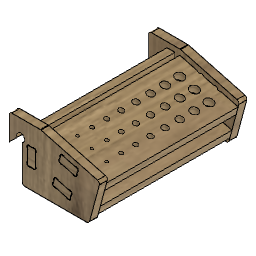
drillbox (Autodesk Fusion 360 design; units mm, degrees)
Autodesk Fusion 360 part; units mm, degrees
note: some values were not read from the file. Set by a fixed rule: which sketch regions a step uses.
sketch "Sketch1" plane through (0, 0, 0) normal (0, 1, 0) x (1, 0, 0) in component "Left"
  line L0 (-26.4881, -75.7327) -> (-26.4881, -48.7327)
  line L1 (-26.4881, -48.7327) -> (-11.4881, -63.7327)
  line L2 (-26.4881, -48.7327) -> (3.3546, -48.7327) construction
  line L3 (-11.4881, -63.7327) -> (-11.4881, -78.7327)
  line L4 (-11.4881, -78.7327) -> (-23.4881, -78.7327)
  line L5 (-11.4881, -78.7327) -> (-11.4881, -16.7327)
  line L6 (-8.4881, -13.7327) -> (-5.4881, -13.7327)
  line L7 (-11.4881, -78.7327) -> (9.1169, -78.7327)
  line L8 (9.8934, -78.6304) -> (74.2289, -61.3918)
  line L9 (9.5119, -78.7327) -> (86.2734, -78.7327) construction
  line L10 (76.3502, -57.7175) -> (65.1603, -15.9562)
  line L11 (62.2625, -13.7327) -> (-5.4881, -13.7327)
  line L12 (64.5645, -13.7327) -> (3.3222, -30.1425)
  arc A0 (74.2289, -61.3918) -> (76.3502, -57.7175) centre (73.4525, -58.494) ccw
  arc A1 (9.1169, -78.7327) -> (9.8934, -78.6304) centre (9.1169, -75.7327) ccw
  arc A2 (-26.4881, -75.7327) -> (-23.4881, -78.7327) centre (-23.4881, -75.7327) ccw
  arc A3 (-8.4881, -13.7327) -> (-11.4881, -16.7327) centre (-8.4881, -16.7327) ccw
  arc A4 (65.1603, -15.9562) -> (62.2625, -13.7327) centre (62.2625, -16.7327) ccw
  point P0 (-26.4881, -78.7327)
  point P1 (-11.4881, -13.7327)
  point P2 (77.1267, -60.6153)
  dimension "d2" = 30
  dimension "d3" = 45
  dimension "d4" = 15
  dimension "d5" = 65
  dimension "d6" = 6
  dimension "d7" = 21
  dimension "d8" = 70
  dimension "d9" = 15
  dimension "d17" = 48.5365
  dimension "d18" = 3
  constraint vertical L0
  constraint horizontal L2
  constraint vertical L3
  constraint perpendicular L0 L4
  constraint perpendicular L2 L5
  constraint perpendicular L5 L6
  constraint perpendicular L3 L7
  constraint horizontal L9
  constraint perpendicular L8 L10
  constraint parallel L6 L11
  constraint parallel L8 L12
  constraint coincident P2 L8
  constraint coincident P2 L10
  constraint tangent L8 A0
  constraint tangent L10 A0
  constraint coincident L9.start L8
  constraint coincident L9.start L7
  constraint tangent L8 A1
  constraint tangent L7 A1
  constraint equal A0 A1
  constraint coincident P0 L0
  constraint coincident P0 L4
  constraint tangent L0 A2
  constraint tangent L4 A2
  constraint equal A0 A2
  constraint coincident P1 L5
  constraint coincident P1 L6
  constraint tangent L5 A3
  constraint tangent L6 A3
  constraint equal A0 A3
  constraint coincident L12.start L11
  constraint coincident L12.start L10
  constraint tangent L11 A4
  constraint tangent L10 A4
  constraint equal A0 A4
  measures "d2" distance of P0 L0.end
  measures "d3" angle of L1 L2
  measures "d4" distance of L0 L1.end
  measures "d5" distance of L3.end P1
  measures "d6" distance of P1 L6.end
  measures "d7" distance of L3.end L9.start
  measures "d8" distance of L9.start P2
  measures "d9" angle of L8 L9
  measures "d17" distance of L8 L12
  measures "d18" radius of A0
extrude "Extrude1" add sketch "Sketch1" along normal blind 9 makes body 1 in component "Left"
sketch "Sketch2" plane through (0, 9, 0) normal (0, 1, 0) x (-1, 0, 0) in component "Deckel"
  line L0 (23.4881, 78.7327) -> (-9.1169, 78.7327)
  line L1 (-9.8934, 78.6304) -> (-74.2289, 61.3918)
  line L2 (-62.2625, 13.7327) -> (8.4881, 13.7327)
  line L3 (11.4881, 16.7327) -> (11.4881, 63.7327)
  line L4 (11.4881, 63.7327) -> (26.4881, 48.7327)
  line L5 (26.4881, 48.7327) -> (26.4881, 75.7327)
  line L6 (-75.5738, 54.8198) -> (-9.1169, 72.6268)
  line L7 (-9.1169, 78.7327) -> (-9.1169, 13.7327) construction
  line L8 (-75.5738, 54.8198) -> (-73.2444, 46.1264)
  line L9 (-73.2444, 46.1264) -> (-6.7876, 63.9335)
  line L10 (-6.7876, 63.9335) -> (-9.1169, 72.6268)
  line L11 (-76.3502, 57.7175) -> (-65.1603, 15.9562)
  arc A0 (-9.1169, 78.7327) -> (-9.8934, 78.6304) centre (-9.1169, 75.7327) ccw
  arc A1 (-74.2289, 61.3918) -> (-76.3502, 57.7175) centre (-73.4525, 58.494) ccw
  arc A2 (-65.1603, 15.9562) -> (-62.2625, 13.7327) centre (-62.2625, 16.7327) ccw
  arc A3 (8.4881, 13.7327) -> (11.4881, 16.7327) centre (8.4881, 16.7327) ccw
  arc A4 (26.4881, 75.7327) -> (23.4881, 78.7327) centre (23.4881, 75.7327) ccw
  line L12 (-76.3502, 57.7175) -> (-65.1603, 15.9562)
  dimension "d12" = 6
  dimension "d14" = 9
  constraint parallel L1 L6
  constraint coincident L0.end L7.start
  constraint coincident L2 L7.end
  constraint perpendicular L2 L7
  constraint coincident L6.end L7
  constraint perpendicular L6 L8
  constraint perpendicular L8 L9
  constraint parallel L8 L10
  constraint collinear L8 L12
  measures "d12" distance of L1 L6
  measures "d14" distance of L6.start L8.end
extrude "Extrude2" add sketch "Sketch2" along normal blind 150 separate body contours L6 L8 L9 L10 L11 L12 makes body 2 in component "Deckel"
ref_plane "WorkPlane1" through (41.1807, 84, 59.3766) normal (0, 1, 0) x (0, 0, 1) in component "Deckel"
mirror "MirrorComponent1" about plane through (0, 0, 0) normal (0, 0, 1) of bodies 1 makes body 3 in component "Right"
sketch "Sketch3" plane through (0, 9, 0) normal (0, 1, 0) x (-1, 0, 0) in component "Boden"
  line L0 (23.4881, 78.7327) -> (-9.1169, 78.7327)
  arc A0 (-9.1169, 78.7327) -> (-9.8934, 78.6304) centre (-9.1169, 75.7327) ccw
  line L1 (-9.8934, 78.6304) -> (-74.2289, 61.3918)
  arc A1 (-74.2289, 61.3918) -> (-76.3502, 57.7175) centre (-73.4525, 58.494) ccw
  line L2 (-76.3502, 57.7175) -> (-65.1603, 15.9562)
  arc A2 (-65.1603, 15.9562) -> (-62.2625, 13.7327) centre (-62.2625, 16.7327) ccw
  line L3 (-62.2625, 13.7327) -> (8.4881, 13.7327)
  arc A3 (8.4881, 13.7327) -> (11.4881, 16.7327) centre (8.4881, 16.7327) ccw
  line L4 (11.4881, 16.7327) -> (11.4881, 63.7327)
  line L5 (11.4881, 63.7327) -> (26.4881, 48.7327)
  line L6 (26.4881, 48.7327) -> (26.4881, 75.7327)
  arc A4 (26.4881, 75.7327) -> (23.4881, 78.7327) centre (23.4881, 75.7327) ccw
  line L7 (-76.3502, 57.7175) -> (-65.1603, 15.9562)
  line L8 (-62.2625, 13.7327) -> (8.4881, 13.7327)
  line L9 (-76.3502, 57.7175) -> (-62.9511, 7.7115) construction
  line L10 (8.4881, 13.7327) -> (-75.9622, 13.7327) construction
  line L11 (-6.7876, 63.9335) -> (-9.1169, 72.6268) construction
  line L12 (-73.2444, 46.1264) -> (-6.7876, 63.9335) construction
  line L13 (-64.5645, 13.7327) -> (1.8923, 31.5397) construction
  line L14 (-66.1174, 19.5282) -> (-68.4468, 28.2215)
  line L15 (-6.7876, 63.9335) -> (-6.7876, 18.0069) construction
  line L16 (-66.1174, 19.5282) -> (-6.7876, 35.4256)
  line L17 (-6.7876, 35.4256) -> (-9.1169, 44.1189)
  line L18 (-9.1169, 44.1189) -> (-68.4468, 28.2215)
  dimension "d22" = 9
  constraint coincident A1.end L2.start
  constraint tangent A1 L9
  constraint parallel L2 L9
  constraint coincident L3.end A3.start
  constraint tangent A3 L10
  constraint parallel L8 L10
  constraint coincident L9 L13.start
  constraint coincident L10 L13.start
  constraint coincident L2 L14.start
  constraint coincident L2 L14.end
  constraint coincident L11.start L12.end
  constraint vertical L15
  constraint coincident L15 L16.end
  constraint perpendicular L7 L16
  constraint perpendicular L14 L18
  measures "d22" distance of L14.start L14.end
extrude "Extrude1'" add sketch "Sketch3" along normal blind 150 separate body contours L2 L7 L14 L16 L17 L18 makes body 4 in component "Boden"
mirror "MirrorComponent2" about plane through (0, 0, 0) normal (0, 0, 1) of bodies 1 makes body 5 in component "Left(Mirror)"
sketch "Sketch1 (2)" plane through (0, 9, 0) normal (0, 1, 0) x (-1, 0, 0) in component "Hinten"
  line L0 (23.4881, 78.7327) -> (-9.1169, 78.7327)
  arc A0 (-9.1169, 78.7327) -> (-9.8934, 78.6304) centre (-9.1169, 75.7327) ccw
  line L1 (-9.8934, 78.6304) -> (-74.2289, 61.3918)
  arc A1 (-74.2289, 61.3918) -> (-76.3502, 57.7175) centre (-73.4525, 58.494) ccw
  line L2 (-76.3502, 57.7175) -> (-65.1603, 15.9562)
  arc A2 (-65.1603, 15.9562) -> (-62.2625, 13.7327) centre (-62.2625, 16.7327) ccw
  line L3 (-62.2625, 13.7327) -> (8.4881, 13.7327)
  arc A3 (8.4881, 13.7327) -> (11.4881, 16.7327) centre (8.4881, 16.7327) ccw
  line L4 (11.4881, 16.7327) -> (11.4881, 63.7327)
  line L5 (11.4881, 63.7327) -> (26.4881, 48.7327)
  line L6 (26.4881, 48.7327) -> (26.4881, 75.7327)
  arc A4 (26.4881, 75.7327) -> (23.4881, 78.7327) centre (23.4881, 75.7327) ccw
  line L7 (5.4881, 19.7327) -> (-3.5119, 19.7327)
  line L8 (-3.5119, 19.7327) -> (-3.5119, 72.7327)
  line L9 (-3.5119, 72.7327) -> (5.4881, 72.7327)
  line L10 (5.4881, 72.7327) -> (5.4881, 19.7327)
  dimension "d26" = 9
  dimension "d27" = 6
  dimension "d28" = 6
  dimension "d29" = 6
  constraint horizontal L7
  constraint vertical L8
  constraint horizontal L9
  constraint vertical L10
  measures "d26" distance of L7.start L7.end
  measures "d27" distance of L3 L7
  measures "d28" distance of L4 L10
  measures "d29" distance of L0 L9
extrude "Extrude1''" add sketch "Sketch1 (2)" along normal blind 150 separate body contours L7 L8 L9 L10 makes body 6 in component "Hinten"
sketch "Sketch1 (3)" plane through (0, 9, 0) normal (0, -1, 0) x (1, 0, 0) in component "Deckel"
  line L0 (6.7876, 63.9335) -> (73.2444, 46.1264)
  line L1 (73.2444, 46.1264) -> (75.5738, 54.8198)
  line L2 (75.5738, 54.8198) -> (9.1169, 72.6268)
  line L3 (9.1169, 72.6268) -> (6.7876, 63.9335)
  line L4 (30.3567, 57.6182) -> (32.6861, 66.3115)
  line L5 (52.0046, 61.1351) -> (49.6752, 52.4418)
  line L6 (49.6752, 52.4418) -> (30.3567, 57.6182)
  line L7 (52.0046, 61.1351) -> (32.6861, 66.3115)
  line L8 (7.9522, 68.2802) -> (31.5214, 61.9648) construction
  line L9 (50.8399, 56.7884) -> (74.4091, 50.4731) construction
  dimension "d32" = 20
  constraint coincident L0 L4.start
  constraint coincident L2 L4.end
  constraint perpendicular L2 L4
  constraint coincident L2 L5.start
  constraint coincident L0 L5.end
  constraint perpendicular L0 L5
  constraint perpendicular L4 L6
  constraint midpoint L3 L8.start
  constraint midpoint L4 L8.end
  constraint midpoint L5 L9.start
  constraint midpoint L1 L9.end
  constraint equal L8 L9
  measures "d32" distance of L4.end L5.start
extrude "Extrude1'''" add sketch "Sketch1 (3)" along normal blind 9 contours L0 L2 L4 L5 L6 L7 bodies 2 in component "Deckel"
sketch "Sketch2 (1)" plane through (0, 159, 0) normal (0, 1, 0) x (-1, 0, 0) in component "Deckel"
  line L0 (-73.2444, 46.1264) -> (-6.7876, 63.9335)
  line L1 (-6.7876, 63.9335) -> (-9.1169, 72.6268)
  line L2 (-9.1169, 72.6268) -> (-75.5738, 54.8198)
  line L3 (-75.5738, 54.8198) -> (-73.2444, 46.1264)
  line L4 (-52.0046, 61.1351) -> (-49.6752, 52.4418)
  line L5 (-30.3567, 57.6182) -> (-32.6861, 66.3115)
  line L6 (-52.0046, 61.1351) -> (-32.6861, 66.3115)
  line L7 (-49.6752, 52.4418) -> (-30.3567, 57.6182)
  line L8 (-50.8399, 56.7884) -> (-74.4091, 50.4731) construction
  line L9 (-31.5214, 61.9648) -> (-7.9522, 68.2802) construction
  dimension "d35" = 20
  constraint coincident L2 L4.start
  constraint coincident L0 L4.end
  constraint perpendicular L0 L4
  constraint coincident L0 L5.start
  constraint coincident L2 L5.end
  constraint perpendicular L2 L5
  constraint midpoint L4 L8.start
  constraint midpoint L3 L8.end
  constraint midpoint L5 L9.start
  constraint midpoint L1 L9.end
  constraint equal L8 L9
  measures "d35" distance of L4.start L5.end
extrude "Extrude2'" add sketch "Sketch2 (1)" along normal blind 9 contours L0 L2 L4 L5 L6 L7 bodies 2 in component "Deckel"
sketch "Sketch3 (2)" plane through (0, 0, 0) normal (0, 1, 0) x (1, 0, 0) in component "Left"
  line L0 (49.6752, -52.4418) -> (52.0046, -61.1351)
  line L1 (52.0046, -61.1351) -> (32.6861, -66.3115)
  line L2 (32.6861, -66.3115) -> (30.3567, -57.6182)
  line L3 (30.3567, -57.6182) -> (49.6752, -52.4418)
  line L4 (30.3567, -57.6182) -> (49.6752, -52.4418)
  line L5 (49.6752, -52.4418) -> (52.0046, -61.1351)
  line L6 (52.0046, -61.1351) -> (32.6861, -66.3115)
  line L7 (32.6861, -66.3115) -> (30.3567, -57.6182)
  constraint coincident L2.end L3.start
  constraint coincident L0.start L3.end
  constraint coincident L0.end L1.start
  constraint coincident L1.end L2.start
extrude "Extrude3" cut sketch "Sketch3 (2)" along normal blind 9 bodies 1 in component "Left"
sketch "Sketch4" plane through (0, 9, 0) normal (0, -1, 0) x (1, 0, 0) in component "Boden"
  line L0 (9.1169, 44.1189) -> (6.7876, 35.4256)
  line L1 (6.7876, 35.4256) -> (66.1174, 19.5282)
  line L2 (66.1174, 19.5282) -> (68.4468, 28.2215)
  line L3 (68.4468, 28.2215) -> (9.1169, 44.1189)
  line L4 (49.6752, 52.4418) -> (52.0046, 61.1351) construction
  line L5 (52.0046, 61.1351) -> (42.5483, 25.8435) construction
  line L6 (42.5483, 25.8435) -> (44.8776, 34.5369)
  line L7 (25.5591, 39.7133) -> (44.8776, 34.5369)
  line L8 (25.5591, 39.7133) -> (23.2298, 31.0199)
  line L9 (23.2298, 31.0199) -> (42.5483, 25.8435)
  dimension "d40" = 20
  constraint coincident L4.end L5.start
  constraint coincident L1 L5.end
  constraint perpendicular L1 L5
  constraint coincident L5 L6.end
  constraint coincident L3 L6.end
  constraint coincident L3 L7.start
  constraint perpendicular L6 L7
  constraint coincident L1 L8.end
  constraint perpendicular L1 L8
  measures "d40" distance of L6.end L7.start
extrude "Extrude2''" add sketch "Sketch4" along normal blind 9 contours L1 L3 L6 L7 L8 L9 bodies 4 in component "Boden"
sketch "Sketch5" plane through (0, 159, 0) normal (0, 1, 0) x (-1, 0, 0) in component "Boden"
  line L0 (-6.7876, 35.4256) -> (-9.1169, 44.1189)
  line L1 (-9.1169, 44.1189) -> (-68.4468, 28.2215)
  line L2 (-68.4468, 28.2215) -> (-66.1174, 19.5282)
  line L3 (-66.1174, 19.5282) -> (-6.7876, 35.4256)
  line L4 (-52.0046, 61.1351) -> (-49.6752, 52.4418)
  line L5 (-52.0046, 61.1351) -> (-42.5483, 25.8435) construction
  line L6 (-44.8776, 34.5369) -> (-42.5483, 25.8435)
  line L7 (-42.5483, 25.8435) -> (-23.2298, 31.0199)
  line L8 (-23.2298, 31.0199) -> (-25.5591, 39.7133)
  line L9 (-25.5591, 39.7133) -> (-44.8776, 34.5369)
  dimension "d43" = 20
  constraint coincident L4.start L5.start
  constraint coincident L3 L5.end
  constraint perpendicular L3 L5
  constraint coincident L5 L6.start
  constraint coincident L1 L6.start
  constraint perpendicular L5 L7
  constraint coincident L1 L8.end
  constraint perpendicular L1 L8
  measures "d43" distance of L5.end L7.end
extrude "Extrude3'" add sketch "Sketch5" along normal blind 9 contours L1 L3 L6 L7 L8 L9 bodies 4 in component "Boden"
sketch "Sketch4 (2)" plane through (0, 0, 0) normal (0, 1, 0) x (1, 0, 0) in component "Left"
  line L0 (25.5591, -39.7133) -> (23.2298, -31.0199)
  line L1 (23.2298, -31.0199) -> (42.5483, -25.8435)
  line L2 (42.5483, -25.8435) -> (44.8776, -34.5369)
  line L3 (44.8776, -34.5369) -> (25.5591, -39.7133)
  line L4 (25.5591, -39.7133) -> (44.8776, -34.5369)
  line L5 (44.8776, -34.5369) -> (42.5483, -25.8435)
  line L6 (42.5483, -25.8435) -> (23.2298, -31.0199)
  line L7 (23.2298, -31.0199) -> (25.5591, -39.7133)
  constraint perpendicular L4 L5
  constraint parallel L4 L6
  constraint parallel L5 L7
  constraint coincident L2.end L3.start
  constraint perpendicular L2 L4
  constraint coincident L0.start L3.end
extrude "Extrude4" cut sketch "Sketch4 (2)" along normal blind 9 bodies 1 in component "Left"
sketch "Sketch2 (2)" plane through (0, 9, 0) normal (0, -1, 0) x (1, 0, 0) in component "Hinten"
  line L0 (3.5119, 72.7327) -> (-5.4881, 72.7327)
  line L1 (-5.4881, 72.7327) -> (-5.4881, 19.7327)
  line L2 (-5.4881, 19.7327) -> (3.5119, 19.7327)
  line L3 (3.5119, 19.7327) -> (3.5119, 72.7327)
  line L4 (-5.4881, 56.2327) -> (3.5119, 56.2327)
  line L5 (3.5119, 56.2327) -> (3.5119, 36.2327)
  line L6 (3.5119, 36.2327) -> (-5.4881, 36.2327)
  line L7 (-5.4881, 36.2327) -> (-5.4881, 56.2327)
  line L8 (-0.9881, 56.2327) -> (-0.9881, 72.7327) construction
  line L9 (-0.9881, 36.2327) -> (-0.9881, 19.7327) construction
  dimension "d48" = 9
  dimension "d49" = 20
  constraint horizontal L4
  constraint vertical L5
  constraint horizontal L6
  constraint vertical L7
  constraint coincident L1 L4.start
  constraint midpoint L4 L8.start
  constraint midpoint L0 L8.end
  constraint midpoint L6 L9.start
  constraint midpoint L2 L9.end
  constraint equal L8 L9
  measures "d48" distance of L4.start L4.end
  measures "d49" distance of L4.start L6.end
extrude "Extrude2'''" add sketch "Sketch2 (2)" along normal blind 9 contours L1 L3 L4 L5 L6 L7 bodies 6 in component "Hinten"
sketch "Sketch3 (3)" plane through (0, 159, 0) normal (0, 1, 0) x (-1, 0, 0) in component "Hinten"
  line L0 (5.4881, 72.7327) -> (-3.5119, 72.7327)
  line L1 (-3.5119, 72.7327) -> (-3.5119, 19.7327)
  line L2 (-3.5119, 19.7327) -> (5.4881, 19.7327)
  line L3 (5.4881, 19.7327) -> (5.4881, 72.7327)
  line L4 (-3.5119, 56.2327) -> (5.4881, 56.2327)
  line L5 (5.4881, 56.2327) -> (5.4881, 36.2327)
  line L6 (5.4881, 36.2327) -> (-3.5119, 36.2327)
  line L7 (-3.5119, 36.2327) -> (-3.5119, 56.2327)
  line L8 (0.9881, 72.7327) -> (0.9881, 56.2327) construction
  line L9 (0.9881, 36.2327) -> (0.9881, 19.7327) construction
  dimension "d52" = 9
  dimension "d53" = 20
  constraint horizontal L4
  constraint vertical L5
  constraint horizontal L6
  constraint vertical L7
  constraint coincident L1 L4.start
  constraint midpoint L0 L8.start
  constraint midpoint L4 L8.end
  constraint midpoint L6 L9.start
  constraint midpoint L2 L9.end
  constraint equal L8 L9
  measures "d52" distance of L4.start L4.end
  measures "d53" distance of L4.start L6.end
extrude "Extrude3''" add sketch "Sketch3 (3)" along normal blind 9 contours L1 L3 L4 L5 L6 L7 bodies 6 in component "Hinten"
sketch "Sketch5 (2)" plane through (0, 0, 0) normal (0, 1, 0) x (1, 0, 0) in component "Left"
  line L0 (-5.4881, -36.2327) -> (3.5119, -36.2327)
  line L1 (3.5119, -36.2327) -> (3.5119, -56.2327)
  line L2 (3.5119, -56.2327) -> (-5.4881, -56.2327)
  line L3 (-5.4881, -56.2327) -> (-5.4881, -36.2327)
extrude "Extrude5" cut sketch "Sketch5 (2)" along normal blind 9 bodies 1 in component "Left"
sketch "Sketch3 (4)" plane through (18.7674, 0, 70.041) normal (0.258819, 0, 0.965926) x (0, 1, 0) in component "Deckel"
  line L0 (9, -34.4097) -> (9, -58.8103)
  line L1 (9, -58.8103) -> (159, -58.8103)
  line L2 (159, -58.8103) -> (159, -34.4097)
  line L3 (159, -34.4097) -> (168, -34.4097)
  line L4 (168, -34.4097) -> (168, -14.4097)
  line L5 (168, -14.4097) -> (159, -14.4097)
  line L6 (159, -14.4097) -> (159, 9.9909)
  line L7 (159, 9.9909) -> (9, 9.9909)
  line L8 (9, 9.9909) -> (9, -14.4097)
  line L9 (9, -14.4097) -> (0, -14.4097)
  line L10 (0, -14.4097) -> (0, -34.4097)
  line L11 (0, -34.4097) -> (9, -34.4097)
  line L12 (0, -24.4097) -> (168, -24.4097) construction
  line L13 (9, -41.61) -> (159, -41.61) construction
  line L14 (9, -7.2094) -> (159, -7.2094) construction
  line L15 (48.2855, -24.4097) -> (48.2855, -7.2094) construction
  line L16 (53.6322, -7.2094) -> (53.6322, 9.9909) construction
  line L17 (66.3625, -24.4097) -> (66.3625, -41.61) construction
  line L18 (72.4731, -41.61) -> (72.4731, -58.8103) construction
  circle A0 centre (142.3333, -41.61) radius 5
  circle A1 centre (125.6667, -41.61) radius 4.5
  circle A2 centre (109, -41.61) radius 4
  circle A3 centre (92.3333, -41.61) radius 3.5
  circle A4 centre (59, -41.61) radius 2.5
  circle A5 centre (42.3333, -41.61) radius 2
  circle A6 centre (25.6667, -41.61) radius 1.5
  circle A7 centre (75.6667, -41.61) radius 3
  circle A8 centre (142.3333, -7.2094) radius 5
  circle A9 centre (125.6667, -7.2094) radius 4.5
  circle A10 centre (109, -7.2094) radius 4
  circle A11 centre (92.3333, -7.2094) radius 3.5
  circle A12 centre (75.6667, -7.2094) radius 3
  circle A13 centre (59, -7.2094) radius 2.5
  circle A14 centre (25.6667, -7.2094) radius 1.5
  circle A15 centre (42.3333, -7.2094) radius 2
  line L19 (9, -33.0098) -> (159.0447, -33.0098) construction
  line L20 (12.5924, -33.0098) -> (12.5924, -24.4097) construction
  line L21 (17.0383, -33.0098) -> (17.0383, -41.61) construction
  circle A16 centre (25.6667, -24.4097) radius 1.5
  circle A17 centre (42.3333, -24.4097) radius 2
  circle A18 centre (59, -24.4097) radius 2.5
  circle A19 centre (75.6667, -24.4097) radius 3
  circle A20 centre (92.3333, -24.4097) radius 3.5
  circle A21 centre (109, -24.4097) radius 4
  circle A22 centre (125.6667, -24.4097) radius 4.5
  circle A23 centre (142.3333, -24.4097) radius 5
  dimension "d59" = 10
  dimension "d60" = 9
  dimension "d61" = 8
  dimension "d62" = 7
  dimension "d64" = 5
  dimension "d65" = 4
  dimension "d66" = 3
  dimension "d67" = 16.6667
  dimension "d68" = 16.6667
  dimension "d69" = 16.6667
  dimension "d71" = 16.6667
  dimension "d72" = 16.6667
  dimension "d73" = 16.6667
  dimension "d74" = 16.6667
  dimension "d75" = 6
  dimension "d76" = 16.6667
  dimension "d77" = 17.2003
  constraint midpoint L10 L12.start
  constraint midpoint L4 L12.end
  constraint coincident L0 L13.start
  constraint coincident L2 L13.end
  constraint perpendicular L2 L13
  constraint coincident L8 L14.start
  constraint coincident L6 L14.end
  constraint perpendicular L6 L14
  constraint coincident L12 L15.start
  constraint coincident L14 L15.end
  constraint perpendicular L14 L15
  constraint coincident L14 L16.start
  constraint coincident L7 L16.end
  constraint perpendicular L7 L16
  constraint equal L15 L16
  constraint coincident L12 L17.start
  constraint coincident L13 L17.end
  constraint perpendicular L13 L17
  constraint coincident L13 L18.start
  constraint coincident L1 L18.end
  constraint perpendicular L1 L18
  constraint equal L17 L18
  constraint coincident L13 A0.centre
  constraint coincident L13 A1.centre
  constraint coincident L13 A2.centre
  constraint coincident L13 A3.centre
  constraint coincident L13 A4.centre
  constraint coincident L13 A5.centre
  constraint coincident L13 A6.centre
  constraint coincident L13 A7.centre
  constraint symmetric L12 A0 A8
  constraint symmetric L12 A1 A9
  constraint symmetric L12 A2 A10
  constraint symmetric L12 A3 A11
  constraint symmetric L12 A4 A13
  constraint symmetric L12 A5 A15
  constraint symmetric L12 A6 A14
  constraint symmetric L12 A7 A12
  constraint perpendicular L15 L19
  constraint coincident L19 L20.start
  constraint coincident L12 L20.end
  constraint perpendicular L12 L20
  constraint coincident L19 L21.start
  constraint coincident L13 L21.end
  constraint perpendicular L13 L21
  constraint equal L20 L21
  constraint symmetric A0 L19 A23
  constraint symmetric A1 L19 A22
  constraint symmetric A2 L19 A21
  constraint symmetric A3 L19 A20
  constraint symmetric A4 L19 A18
  constraint symmetric A5 L19 A17
  constraint symmetric A6 L19 A16
  constraint symmetric A7 L19 A19
  measures "d59" diameter of A0
  measures "d60" diameter of A1
  measures "d61" diameter of A2
  measures "d62" diameter of A3
  measures "d64" diameter of A4
  measures "d65" diameter of A5
  measures "d66" diameter of A6
  measures "d67" distance of L0 A6.centre
  measures "d68" distance of A5.centre A6.centre
  measures "d69" distance of A4.centre A5.centre
  measures "d71" distance of L13.end A0.centre
  measures "d72" distance of A0.centre A1.centre
  measures "d73" distance of A1.centre A2.centre
  measures "d74" distance of A2.centre A3.centre
  measures "d75" diameter of A7
  measures "d76" distance of A3.centre A7.centre
  measures "d77" distance of L12 L13
extrude "Extrude3'''" cut sketch "Sketch3 (4)" against normal blind 9 contours A0 | A1 | A2 | A3 | A4 | A5 | A6 | A7 | A8 | A9 | A10 | A11 | A12 | A13 | A14 | A15 | A16 | A17 | A18 | A19 | A20 | A21 | A22 | A23 bodies 2 in component "Deckel"
sketch "dogbone" plane through (0, 0, 0) normal (0, -1, 0) x (-1, 0, 0) in component "Left"
  line L0 (5.4881, -36.2327) -> (5.4881, -56.2327)
  line L1 (5.4881, -56.2327) -> (-3.5119, -56.2327)
  line L2 (-3.5119, -56.2327) -> (-3.5119, -36.2327)
  line L3 (-3.5119, -36.2327) -> (5.4881, -36.2327)
  line L4 (-42.5483, -25.8435) -> (-23.2298, -31.0199)
  line L5 (-23.2298, -31.0199) -> (-25.5591, -39.7133)
  line L6 (-25.5591, -39.7133) -> (-44.8776, -34.5369)
  line L7 (-44.8776, -34.5369) -> (-42.5483, -25.8435)
  line L8 (-30.3567, -57.6182) -> (-32.6861, -66.3115)
  line L9 (-32.6861, -66.3115) -> (-52.0046, -61.1351)
  line L10 (-52.0046, -61.1351) -> (-49.6752, -52.4418)
  line L11 (-49.6752, -52.4418) -> (-30.3567, -57.6182)
  line L12 (-9.1169, -78.7327) -> (23.4881, -78.7327)
  arc A0 (23.4881, -78.7327) -> (26.4881, -75.7327) centre (23.4881, -75.7327) ccw
  line L13 (26.4881, -75.7327) -> (26.4881, -48.7327)
  line L14 (26.4881, -48.7327) -> (11.4881, -63.7327)
  line L15 (11.4881, -63.7327) -> (11.4881, -16.7327)
  arc A1 (11.4881, -16.7327) -> (8.4881, -13.7327) centre (8.4881, -16.7327) ccw
  line L16 (8.4881, -13.7327) -> (-62.2625, -13.7327)
  arc A2 (-62.2625, -13.7327) -> (-65.1603, -15.9562) centre (-62.2625, -16.7327) ccw
  line L17 (-65.1603, -15.9562) -> (-76.3502, -57.7175)
  arc A3 (-76.3502, -57.7175) -> (-74.2289, -61.3918) centre (-73.4525, -58.494) ccw
  line L18 (-74.2289, -61.3918) -> (-9.8934, -78.6304)
  arc A4 (-9.8934, -78.6304) -> (-9.1169, -78.7327) centre (-9.1169, -75.7327) ccw
  point P0 (3.3668, -38.354)
  point P1 (3.3668, -54.1113)
  point P2 (-1.3906, -38.354)
  point P3 (-1.3906, -54.1113)
  point P4 (-41.0483, -28.4416)
  point P5 (-25.8278, -32.5199)
  point P6 (-42.2796, -33.0369)
  point P7 (-27.0591, -37.1152)
  point P8 (-32.9548, -59.1182)
  point P9 (-34.1861, -63.7134)
  point P10 (-48.1752, -55.0398)
  point P11 (-49.4065, -59.6351)
hole "Hole1" at (-3.3668, 0, 38.354) at (-3.3668, 0, 54.1113) at (1.3906, 0, 38.354) at (1.3906, 0, 54.1113) at (41.0483, 0, 28.4416) at (25.8278, 0, 32.5199) at (42.2796, 0, 33.0369) at (27.0591, 0, 37.1152) at (32.9548, 0, 59.1182) at (34.1861, 0, 63.7134) at (48.1752, 0, 55.0398) at (49.4065, 0, 59.6351) direction (0, 1, 0) diameter 6 depth 9 tip angle 180 bodies 1 in component "Left"
sketch "dogbone (2)" plane through (18.7674, 0, 70.041) normal (0.258819, 0, 0.965926) x (0.965926, 0, -0.258819) in component "Deckel"
  circle A0 centre (24.4097, 125.6667) radius 4.5
  circle A1 centre (7.2094, 75.6667) radius 3
  circle A2 centre (7.2094, 42.3333) radius 2
  circle A3 centre (41.61, 42.3333) radius 2
  circle A4 centre (41.61, 92.3333) radius 3.5
  circle A5 centre (24.4097, 142.3333) radius 5
  circle A6 centre (41.61, 142.3333) radius 5
  circle A7 centre (41.61, 75.6667) radius 3
  circle A8 centre (41.61, 25.6667) radius 1.5
  circle A9 centre (7.2094, 59) radius 2.5
  circle A10 centre (7.2094, 92.3333) radius 3.5
  circle A11 centre (7.2094, 125.6667) radius 4.5
  circle A12 centre (24.4097, 109) radius 4
  circle A13 centre (24.4097, 75.6667) radius 3
  circle A14 centre (7.2094, 25.6667) radius 1.5
  circle A15 centre (24.4097, 42.3333) radius 2
  circle A16 centre (41.61, 109) radius 4
  circle A17 centre (7.2094, 142.3333) radius 5
  circle A18 centre (41.61, 125.6667) radius 4.5
  circle A19 centre (41.61, 59) radius 2.5
  circle A20 centre (24.4097, 25.6667) radius 1.5
  circle A21 centre (24.4097, 59) radius 2.5
  circle A22 centre (24.4097, 92.3333) radius 3.5
  circle A23 centre (7.2094, 109) radius 4
  line L0 (34.4097, 9) -> (58.8103, 9)
  line L1 (58.8103, 9) -> (58.8103, 159)
  line L2 (58.8103, 159) -> (34.4097, 159)
  line L3 (34.4097, 159) -> (34.4097, 168)
  line L4 (34.4097, 168) -> (14.4097, 168)
  line L5 (14.4097, 168) -> (14.4097, 159)
  line L6 (14.4097, 159) -> (-9.9909, 159)
  line L7 (-9.9909, 159) -> (-9.9909, 9)
  line L8 (-9.9909, 9) -> (14.4097, 9)
  line L9 (14.4097, 9) -> (14.4097, 0)
  line L10 (14.4097, 0) -> (34.4097, 0)
  line L11 (34.4097, 0) -> (34.4097, 9)
  point P0 (12.2883, 161.1213)
  point P1 (36.531, 161.1213)
  point P2 (12.2883, 6.8787)
  point P3 (36.531, 6.8787)
hole "Hole1'" at (30.6371, 161.1213, 66.8605) direction (-0.258819, 0, -0.965926) diameter 6 depth 9 tip angle 180 bodies 2 in component "Deckel"
hole "Hole2" at (54.0536, 161.1213, 60.5861) at (30.6371, 6.8787, 66.8605) direction (-0.258819, 0, -0.965926) diameter 6 depth 9 tip angle 180 bodies 2 in component "Deckel"
hole "Hole3" at (54.0536, 6.8787, 60.5861) direction (-0.258819, 0, -0.965926) diameter 6 depth 9 tip angle 180 bodies 2 in component "Deckel"
sketch "dogbone (3)" plane through (11.6405, 0, 43.4428) normal (0.258819, 0, 0.965926) x (0.965926, 0, -0.258819) in component "Boden"
  line L0 (-2.6125, 9) -> (14.4097, 9)
  line L1 (14.4097, 9) -> (14.4097, 0)
  line L2 (14.4097, 0) -> (34.4097, 0)
  line L3 (34.4097, 0) -> (34.4097, 9)
  line L4 (34.4097, 9) -> (58.8103, 9)
  line L5 (58.8103, 9) -> (58.8103, 159)
  line L6 (58.8103, 159) -> (34.4097, 159)
  line L7 (34.4097, 159) -> (34.4097, 168)
  line L8 (34.4097, 168) -> (14.4097, 168)
  line L9 (14.4097, 168) -> (14.4097, 159)
  line L10 (14.4097, 159) -> (-2.6125, 159)
  line L11 (-2.6125, 159) -> (-2.6125, 9)
  point P0 (12.2883, 161.1213)
  point P1 (36.531, 161.1213)
  point P2 (36.531, 6.8787)
  point P3 (12.2883, 6.8787)
hole "Hole1''" at (23.5101, 161.1213, 40.2623) direction (-0.258819, 0, -0.965926) diameter 6 depth 9 tip angle 180 bodies 4 in component "Boden"
hole "Hole2'" at (46.9267, 161.1213, 33.9878) direction (-0.258819, 0, -0.965926) diameter 6 depth 9 tip angle 180 bodies 4 in component "Boden"
hole "Hole3'" at (23.5101, 6.8787, 40.2623) direction (-0.258819, 0, -0.965926) diameter 6 depth 9 tip angle 180 bodies 4 in component "Boden"
hole "Hole4" at (46.9267, 6.8787, 33.9878) direction (-0.258819, 0, -0.965926) diameter 6 depth 9 tip angle 180 bodies 4 in component "Boden"
sketch "dogbone (4)" plane through (-5.4881, 0, 0) normal (-1, 0, 0) x (0, 0, 1) in component "Hinten"
  line L0 (56.2327, 9) -> (72.7327, 9)
  line L1 (72.7327, 9) -> (72.7327, 159)
  line L2 (72.7327, 159) -> (56.2327, 159)
  line L3 (56.2327, 159) -> (56.2327, 168)
  line L4 (56.2327, 168) -> (36.2327, 168)
  line L5 (36.2327, 168) -> (36.2327, 159)
  line L6 (36.2327, 159) -> (19.7327, 159)
  line L7 (19.7327, 159) -> (19.7327, 9)
  line L8 (19.7327, 9) -> (36.2327, 9)
  line L9 (36.2327, 9) -> (36.2327, 0)
  line L10 (36.2327, 0) -> (56.2327, 0)
  line L11 (56.2327, 0) -> (56.2327, 9)
  point P0 (58.354, 161.1213)
  point P1 (34.1113, 161.1213)
  point P2 (58.354, 6.8787)
  point P3 (34.1113, 6.8787)
hole "Hole1'''" at (-5.4881, 161.1213, 58.354) at (-5.4881, 161.1213, 34.1113) at (-5.4881, 6.8787, 58.354) at (-5.4881, 6.8787, 34.1113) direction (1, 0, 0) diameter 6 depth 9 tip angle 180 bodies 6 in component "Hinten"
sketch "dogbone (1)" plane through (0, 0, 0) normal (0, -1, 0) x (-1, 0, 0) in component "Left"
  arc A0 (-50.9065, -57.037) -> (-47.9065, -62.2332) centre (-49.4065, -59.6351) ccw
  line L0 (-50.9065, -57.037) -> (-50.7733, -56.5398)
  arc A1 (-45.5772, -53.5398) -> (-50.7733, -56.5398) centre (-48.1752, -55.0398) ccw
  line L1 (-45.5772, -53.5398) -> (-34.4548, -56.5201)
  arc A2 (-31.4548, -61.7162) -> (-34.4548, -56.5201) centre (-32.9548, -59.1182) ccw
  line L2 (-31.4548, -61.7162) -> (-31.588, -62.2134)
  arc A3 (-36.7842, -65.2134) -> (-31.588, -62.2134) centre (-34.1861, -63.7134) ccw
  line L3 (-36.7842, -65.2134) -> (-47.9065, -62.2332)
  arc A4 (-43.7796, -30.4388) -> (-40.7796, -35.635) centre (-42.2796, -33.0369) ccw
  line L4 (-43.7796, -30.4388) -> (-43.6463, -29.9416)
  arc A5 (-38.4502, -26.9416) -> (-43.6463, -29.9416) centre (-41.0483, -28.4416) ccw
  line L5 (-38.4502, -26.9416) -> (-27.3278, -29.9219)
  arc A6 (-24.3278, -35.118) -> (-27.3278, -29.9219) centre (-25.8278, -32.5199) ccw
  line L6 (-24.3278, -35.118) -> (-24.461, -35.6152)
  arc A7 (-29.6572, -38.6152) -> (-24.461, -35.6152) centre (-27.0591, -37.1152) ccw
  line L7 (-29.6572, -38.6152) -> (-40.7796, -35.635)
  arc A8 (0.7308, -36.2327) -> (-3.5119, -40.4753) centre (-1.3906, -38.354) ccw
  line L8 (0.7308, -36.2327) -> (1.2455, -36.2327)
  arc A9 (5.4881, -40.4753) -> (1.2455, -36.2327) centre (3.3668, -38.354) ccw
  line L9 (5.4881, -40.4753) -> (5.4881, -51.99)
  arc A10 (1.2455, -56.2327) -> (5.4881, -51.99) centre (3.3668, -54.1113) ccw
  line L10 (1.2455, -56.2327) -> (0.7308, -56.2327)
  arc A11 (-3.5119, -51.99) -> (0.7308, -56.2327) centre (-1.3906, -54.1113) ccw
  line L11 (-3.5119, -51.99) -> (-3.5119, -40.4753)
  line L12 (-9.1169, -78.7327) -> (23.4881, -78.7327)
  arc A12 (23.4881, -78.7327) -> (26.4881, -75.7327) centre (23.4881, -75.7327) ccw
  line L13 (26.4881, -75.7327) -> (26.4881, -48.7327)
  line L14 (26.4881, -48.7327) -> (11.4881, -63.7327)
  line L15 (11.4881, -63.7327) -> (11.4881, -16.7327)
  arc A13 (11.4881, -16.7327) -> (8.4881, -13.7327) centre (8.4881, -16.7327) ccw
  line L16 (8.4881, -13.7327) -> (-62.2625, -13.7327)
  arc A14 (-62.2625, -13.7327) -> (-65.1603, -15.9562) centre (-62.2625, -16.7327) ccw
  line L17 (-65.1603, -15.9562) -> (-76.3502, -57.7175)
  arc A15 (-76.3502, -57.7175) -> (-74.2289, -61.3918) centre (-73.4525, -58.494) ccw
  line L18 (-74.2289, -61.3918) -> (-9.8934, -78.6304)
  arc A16 (-9.8934, -78.6304) -> (-9.1169, -78.7327) centre (-9.1169, -75.7327) ccw
  point P0 (13.2102, -59.5752)
hole "Hole2''" at (-13.2102, 0, 59.5752) direction (0, 1, 0) diameter 9 depth 9 tip angle 180 bodies 1 in component "Left"
mirror "MirrorComponent3" about plane through (0, 0, 0) normal (0, 0, 1) of bodies 1 makes body 7 in component "Left(Mirror) (1)"
copy_body "CopyPasteBodies3" bodies 1 makes body 8 in component "Cam Layout"
move_body "Move2" bodies 8 to x (1, 0, 0) y (0, 0, 1) z (0, -1, 0) at (0, 13.7327, 13.7327) in component "Cam Layout"
copy_body "CopyPasteBodies4" bodies 2 makes body 9 in component "Cam Layout"
move_body "Move3" bodies 9 to x (0.965926, 0, 0.258819) y (0, 1, 0) z (-0.258819, 0, 0.965926) at (12.1697, 0, -0.185) in component "Cam Layout"
copy_body "CopyPasteBodies5" bodies 4 makes body 10 in component "Cam Layout"
move_body "Move4" bodies 10 to x (0.965926, 0, 0.258819) y (0, 1, 0) z (-0.258819, 0, 0.965926) at (5.2856, 0, -1.0913) in component "Cam Layout"
copy_body "CopyPasteBodies6" bodies 6 makes body 11 in component "Cam Layout"
move_body "Move5" bodies 11 to x (0, 0, 1) y (0, 1, 0) z (-1, 0, 0) at (14.2445, 0, 25.2208) in component "Cam Layout"
copy_body "CopyPasteBodies7" bodies 7 body 7 seen with x (1, 0, 0) y (0, -1, 0) z (0, 0, -1) at (0, 168, 0) makes body 12 in component "Cam Layout"
move_body "Move6" bodies 12 to x (1, 0, 0) y (0, 0, 1) z (0, -1, 0) at (0, 172.7327, -145.2673) in component "Cam Layout"
move_body "Move7" bodies 9 to x (1, 0, 0) y (0, 1, 0) z (0, 0, 1) at (70, 0, 0) in component "Cam Layout"
move_body "Move8" bodies 12 to x (1, 0, 0) y (0, 1, 0) z (0, 0, 1) at (0, 80, 0) in component "Cam Layout"
move_body "Align1" bodies 8 to x (1, 0, 0) y (0, 1, 0) z (0, 0, 1) at (0, 0, 0) in component "Cam Layout"
move_body "Align2" bodies 8 to x (1, 0, 0) y (0, 1, 0) z (0, 0, 1) at (0, 0, 6) in component "Cam Layout"
move_body "Align3" bodies 10 to x (1, 0, 0) y (0, 1, 0) z (0, 0, 1) at (0, 0, -15.1513) in component "Cam Layout"
move_body "Align4" bodies 9 to x (1, 0, 0) y (0, 1, 0) z (0, 0, 1) at (0, 0, -43.5941) in component "Cam Layout"
move_body "Align5" bodies 10 to x (1, 0, 0) y (0, 1, 0) z (0, 0, 1) at (0, 0, -19.7327) in component "Cam Layout"
move_body "Align6" bodies 11 to x (1, 0, 0) y (0, 1, 0) z (0, 0, 1) at (0, 0, -19.7327) in component "Cam Layout"
move_body "Align7" bodies 8 to x (1, 0, 0) y (0, 1, 0) z (0, 0, 1) at (0, 0, -19.7327) in component "Cam Layout"
move_body "Align8" bodies 12 to x (1, 0, 0) y (0, 1, 0) z (0, 0, 1) at (0, 0, -13.7327) in component "Cam Layout"
move_body "Align9" bodies 9 to x (1, 0, 0) y (0, 1, 0) z (0, 0, 1) at (0, 0, -19.7327) in component "Cam Layout"
move_body "Move9" bodies 8 to x (1, 0, 0) y (0, 1, 0) z (0, 0, 1) at (0, -10, 0) in component "Cam Layout"
move_body "Align10" bodies 8 to x (1, 0, 0) y (0, 1, 0) z (0, 0, 1) at (-32, 0, 0) in component "Cam Layout"
move_body "Move10" bodies 12 to x (-1, 0, 0) y (0, -1, 0) z (0, 0, 1) at (127.0238, 167, 0) in component "Cam Layout"
move_body "Move11" bodies 12 to x (1, 0, 0) y (0, 1, 0) z (0, 0, 1) at (-5, 0, 0) in component "Cam Layout"
move_body "Move12" bodies 8 to x (1, 0, 0) y (0, 1, 0) z (0, 0, 1) at (0, 4, 0) in component "Cam Layout"
move_body "Move13" bodies 8 to x (1, 0, 0) y (0, 1, 0) z (0, 0, 1) at (0, -1, 0) in component "Cam Layout"
move_body "Move14" bodies 10 to x (1, 0, 0) y (0, 1, 0) z (0, 0, 1) at (-1.161, 0, 0) in component "Cam Layout"
move_body "Move15" bodies 9 to x (1, 0, 0) y (0, 1, 0) z (0, 0, 1) at (-2.244, 0, 0) in component "Cam Layout"
move_body "Move16" bodies 8 to x (1, 0, 0) y (0, 1, 0) z (0, 0, 1) at (200, 0, 0) in component "Cam Layout"
move_body "Move17" bodies 12 to x (1, 0, 0) y (0, 1, 0) z (0, 0, 1) at (-105, 0, 0) in component "Cam Layout"
move_body "Move18" bodies 8 to x (1, 0, 0) y (0, 1, 0) z (0, 0, 1) at (-100, 0, 0) in component "Cam Layout"
move_body "Move20" bodies 8 to x (1, 0, 0) y (0, 1, 0) z (0, 0, 1) at (-6, 0, 0) in component "Cam Layout"
component "Construction" placed x (1, 0, 0) y (0, 1, 0) z (0, 0, 1) at (0, 0, 0)
component "Cam Layout" placed x (1, 0, 0) y (0, 1, 0) z (0, 0, 1) at (0, 0, 0)
component "Left" placed x (1, 0, 0) y (0, 1, 0) z (0, 0, 1) at (0, 0, 0) in component "Construction"
component "Deckel" placed x (1, 0, 0) y (0, 1, 0) z (0, 0, 1) at (0, 0, 0) in component "Construction"
component "Boden" placed x (1, 0, 0) y (0, 1, 0) z (0, 0, 1) at (0, 0, 0) in component "Construction"
component "Hinten" placed x (1, 0, 0) y (0, 1, 0) z (0, 0, 1) at (0, 0, 0) in component "Construction"
component "Left(Mirror) (1)" placed x (1, 0, 0) y (0, -1, 0) z (0, 0, -1) at (0, 168, 0) in component "Construction"
equation "thickness = 9 mm"
equation "d7 = 6 mm + 9 mm + 6 mm"
equation "d10 = thickness"
equation "d14 = thickness"
equation "d15 = breite"
equation "d18 = fillet"
equation "fillet = 3 mm"
equation "d22 = thickness"
equation "d23 = breite"
equation "breite = 150 mm"
equation "d26 = thickness"
equation "d30 = breite"
equation "d33 = thickness"
equation "d36 = thickness"
equation "d38 = thickness"
equation "d41 = thickness"
equation "d44 = thickness"
equation "d46 = thickness"
equation "d48 = thickness"
equation "d50 = thickness"
equation "d52 = thickness"
equation "d54 = thickness"
equation "d56 = thickness"
equation "d67 = breite / 9"
equation "d68 = breite / 9"
equation "d69 = breite / 9"
equation "d71 = breite / 9"
equation "d72 = breite / 9"
equation "d73 = breite / 9"
equation "d74 = breite / 9"
equation "d76 = breite / 9"
equation "d78 = -thickness"
equation "HoleDepth = 9.00 mm"
equation "HoleDiameter = 6.00 mm"
equation "TipAngle = 180 deg"
